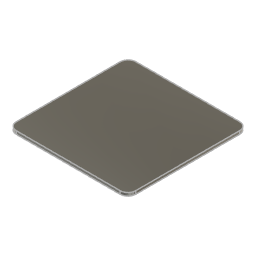
plate (Autodesk Fusion 360 design; units mm, degrees)
Autodesk Fusion 360 part; units mm, degrees
sketch "Sketch1" plane through (0, 0, 0) normal (0, 0, 1) x (1, 0, 0)
  line L0 (0, 0) -> (-70, 0)
  line L1 (-70, 0) -> (-70, -50.9434)
  line L2 (-70, -50.9434) -> (0, -50.9434)
  line L3 (0, -50.9434) -> (0, 0)
  dimension "d1" = 70
  constraint horizontal L0
  constraint vertical L1
  constraint horizontal L2
  constraint vertical L3
  constraint coincident L0.start L3.end
  measures "d1" distance of L0.start L0.end
sketch "Sketch2" plane through (0, 0, 0) normal (0, 0, 1) x (1, 0, 0)
  line L0 (0, 0) -> (76.2, 0)
  line L1 (76.2, 0) -> (76.2, 76.2952)
  line L2 (76.2, 76.2952) -> (0, 76.2952)
  line L3 (0, 76.2952) -> (0, 0)
  dimension "d4" = 76.2
  constraint horizontal L0
  constraint vertical L1
  constraint horizontal L2
  constraint vertical L3
  constraint coincident L0.start L3.end
  measures "d4" distance of L0.start L0.end
extrude "Extrude2" add sketch "Sketch2" along normal blind 2
fillet "Fillet1" radius 5 4 edges at (0, 76.2952, 1) (76.2, 76.2952, 1) (0, 0, 1) (76.2, 0, 1)
